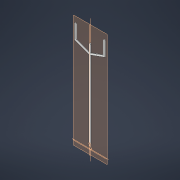
# Autodesk Inventor part: card holder
Saved by Autodesk Inventor 2021 (Build 250183000, 183)
## iProperties
Created: 2020-09-17
Part Number: card holder
Material: Generic
Document SubType Name: Modeling
Designer: brand
Density: 1 g/cm^3
Appearance: Default
Author: brand
Autodesk Inventor part; units mm, degrees
sketch "Sketch1" plane through (0, 0, 0) normal (0, 0, 1) x (1, 0, 0)
  line L0 (0, 0) -> (-2, 15)
  line L1 (-2, 15) -> (-2, 216.3683)
  line L2 (-48, 0) -> (8, 0) projected
  line L3 (-2, 216.3683) -> (-40, 230.1992)
  line L4 (-40, 230.1992) -> (-40, 268)
  line L5 (-40, 268) -> (-38, 270)
  line L6 (-38, 270) -> (-36, 268)
  line L7 (-36, 268) -> (-36, 233)
  line L8 (-36, 233) -> (-2, 220.625)
  line L9 (-2, 220.625) -> (-2, 240.625)
  line L10 (-2, 240.625) -> (0, 242.625)
  line L11 (0, 242.625) -> (0, 0)
  dimension "d6" = 15
  dimension "d7" = 4
  dimension "d12" = 4
  dimension "d19" = 2
  dimension "d20" = 270
  dimension "d22" = 135
  dimension "d23" = 2
  dimension "d24" = 70
  dimension "d26" = 2
  dimension "d27" = 40
  dimension "d28" = 135
  dimension "d31" = 35
  dimension "d32" = 20
  constraints: 22 end point, 3 vertical, 2 parallel, 2 perpendicular, 1 coincident
  measures "d6" distance from line of L2 L0.end
  measures "d7" distance between parallel lines of L7 L4
  measures "d12" distance between parallel lines of L3 L8
  measures "d19" horizontal distance of L4.end L5.end
  measures "d20" distance from line of L2 L5.end
  measures "d22" angle of L9 L10
  measures "d23" distance between parallel lines of L11 L9
  measures "d24" angle of L9 L8
  measures "d26" distance between parallel lines of L11 L1
  measures "d27" distance between parallel lines of L11 L4
  measures "d28" angle of L4 L5
  measures "d31" distance of L6.end L7.end
  measures "d32" distance of L8.end L9.end
extrude "Extrusion1" add sketch "Sketch1" along normal blind 2
mirror "Mirror1" about plane through (0, 0, 0) normal (1, 0, 0) of "Extrusion1"
ref_plane "Work Plane1" through (2, 15, 2) normal (0, -0.1321637, 0.9912279) x (-1, 0, 0)
sketch "Sketch3" plane through (2, 15, 2) normal (0, -0.1321637, 0.9912279) x (-1, 0, 0)
  line L0 (4, -199.6019) -> (4, 0) projected
  line L1 (4, 0) -> (0, 0)
  line L2 (0, 0) -> (0, 15.1327)
  line L3 (0, 15.1327) -> (4, 15.1327)
  line L4 (4, 15.1327) -> (4, 0)
  point P0 (2, 15.1327)
  constraints: 8 end point, 2 parallel, 1 horizontal, 1 midpoint, 1 perpendicular
extrude "Extrusion2" cut sketch "Sketch3" along normal through all
equation "\"d7\" = thickness"
equation "\"d12\" = thickness"
equation "\"d20\" = length"
equation "\"d23\" = 0.5 * thickness"
equation "\"d26\" = 0.5 * thickness"
equation "\"thickness\" = 4"
equation "\"length\" = 270"
body "Solid1"
